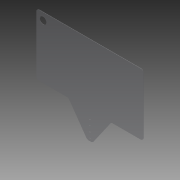
# Autodesk Inventor part: Funnel 2
Saved by Autodesk Inventor 2014 (Build 180170000, 170)
## iProperties
Created: 2014-01-07
Part Number: Funnel 2
Material: Polycarbonate, Clear
Document SubType Name: Modeling
Designer: Michael
Density: 1.2 g/cm^3
Appearance: Polycarbonate - Clear
Author: Michael
Autodesk Inventor part; units mm, degrees
ref_plane "YZ Plane" through (0, 0, 0) normal (1, 0, 0) x (0, 1, 0)
ref_plane "XZ Plane" through (0, 0, 0) normal (0, 1, 0) x (-1, 0, 0)
ref_plane "XY Plane" through (0, 0, 0) normal (0, 0, 1) x (1, 0, 0)
sketch "Sketch1" plane through (0, 0, 0) normal (0, 0, 1) x (1, 0, 0)
  line L0 (0, 0) -> (25.4, 0)
  line L1 (25.4, 0) -> (114.3, 127)
  line L2 (12.7, 0) -> (12.7, 419.1) construction
  line L3 (114.3, 127) -> (266.7, 127)
  line L4 (266.7, 127) -> (266.7, 419.1)
  line L5 (266.7, 419.1) -> (12.7, 419.1)
  circle A0 centre (12.7, 12.7) radius 2.0828
  circle A1 centre (12.7, 38.1) radius 2.0828
  circle A2 centre (12.7, 63.5) radius 2.0828
  circle A3 centre (12.7, 88.9) radius 2.0828
  line L6 (0, 0) -> (-88.9, 127)
  line L7 (-88.9, 127) -> (-241.3, 127)
  line L8 (-241.3, 127) -> (-241.3, 419.1)
  line L9 (-241.3, 419.1) -> (12.7, 419.1)
  dimension "d0" = 25.4
  dimension "d2" = 254
  dimension "d3" = 419.1
  dimension "d4" = 127
  dimension "d5" = 152.4
  dimension "d6" = 4.1656
  dimension "d7" = 12.7
  dimension "d10" = 25.4
  constraints: 20 end point, 4 centre point, 4 perpendicular, 3 symmetric about line, 1 horizontal, 1 midpoint, 1 point on line, 1 vertical, 6 other
  measures "d0" distance of L0.start L0.end
  measures "d2" distance between parallel lines of L2 L4
  measures "d3" distance from line of L2.start L5
  measures "d4" distance between parallel lines of L0 L3
  measures "d5" distance of L1.end L3.end
  measures "d6" diameter of A0
  measures "d7" distance from line of L0 A0.centre
  measures "d10" distance of A0.centre A1.centre
extrude "Extrusion1" add sketch "Sketch1" along normal blind 1.5875
fillet "Fillet1" radius 12.7 8 edges at (25.4, 0, 0.7937) (114.3, 127, 0.7937) (266.7, 127, 0.7937) (266.7, 419.1, 0.7937) (-241.3, 419.1, 0.7937) (-241.3, 127, 0.7937) (-88.9, 127, 0.7937) (0, 0, 0.7937)
sketch "Sketch2" plane through (0, 0, 1.5875) normal (0, 0, 1) x (1, 0, 0)
  line L0 (254, 419.1) -> (-228.6, 419.1) projected
  line L1 (-241.3, 406.4) -> (-241.3, 139.7) projected
  circle A0 centre (-209.55, 384.175) radius 15.875
  circle A1 centre (-165.1, 384.175) radius 15.875
  circle A2 centre (-120.65, 384.175) radius 15.875
  circle A3 centre (-76.2, 384.175) radius 15.875
  circle A4 centre (-31.75, 384.175) radius 15.875
  circle A5 centre (12.7, 384.175) radius 15.875
  circle A6 centre (57.15, 384.175) radius 15.875
  circle A7 centre (101.6, 384.175) radius 15.875
  circle A8 centre (146.05, 384.175) radius 15.875
  circle A9 centre (190.5, 384.175) radius 15.875
  circle A10 centre (234.95, 384.175) radius 15.875
  circle A11 centre (-209.55, 339.725) radius 15.875
  circle A12 centre (-165.1, 339.725) radius 15.875
  circle A13 centre (-120.65, 339.725) radius 15.875
  circle A14 centre (-76.2, 339.725) radius 15.875
  circle A15 centre (-31.75, 339.725) radius 15.875
  circle A16 centre (12.7, 339.725) radius 15.875
  circle A17 centre (57.15, 339.725) radius 15.875
  circle A18 centre (101.6, 339.725) radius 15.875
  circle A19 centre (146.05, 339.725) radius 15.875
  circle A20 centre (190.5, 339.725) radius 15.875
  circle A21 centre (234.95, 339.725) radius 15.875
  circle A22 centre (-209.55, 295.275) radius 15.875
  circle A23 centre (-165.1, 295.275) radius 15.875
  circle A24 centre (-120.65, 295.275) radius 15.875
  circle A25 centre (-76.2, 295.275) radius 15.875
  circle A26 centre (-31.75, 295.275) radius 15.875
  circle A27 centre (12.7, 295.275) radius 15.875
  circle A28 centre (57.15, 295.275) radius 15.875
  circle A29 centre (101.6, 295.275) radius 15.875
  circle A30 centre (146.05, 295.275) radius 15.875
  circle A31 centre (190.5, 295.275) radius 15.875
  circle A32 centre (234.95, 295.275) radius 15.875
  circle A33 centre (-209.55, 250.825) radius 15.875
  circle A34 centre (-165.1, 250.825) radius 15.875
  circle A35 centre (-120.65, 250.825) radius 15.875
  circle A36 centre (-76.2, 250.825) radius 15.875
  circle A37 centre (-31.75, 250.825) radius 15.875
  circle A38 centre (12.7, 250.825) radius 15.875
  circle A39 centre (57.15, 250.825) radius 15.875
  circle A40 centre (101.6, 250.825) radius 15.875
  circle A41 centre (146.05, 250.825) radius 15.875
  circle A42 centre (190.5, 250.825) radius 15.875
  circle A43 centre (234.95, 250.825) radius 15.875
  circle A44 centre (-209.55, 206.375) radius 15.875
  circle A45 centre (-165.1, 206.375) radius 15.875
  circle A46 centre (-120.65, 206.375) radius 15.875
  circle A47 centre (-76.2, 206.375) radius 15.875
  circle A48 centre (-31.75, 206.375) radius 15.875
  circle A49 centre (12.7, 206.375) radius 15.875
  circle A50 centre (57.15, 206.375) radius 15.875
  circle A51 centre (101.6, 206.375) radius 15.875
  circle A52 centre (146.05, 206.375) radius 15.875
  circle A53 centre (190.5, 206.375) radius 15.875
  circle A54 centre (234.95, 206.375) radius 15.875
  circle A55 centre (-209.55, 161.925) radius 15.875
  circle A56 centre (-165.1, 161.925) radius 15.875
  circle A57 centre (-120.65, 161.925) radius 15.875
  circle A58 centre (-76.2, 161.925) radius 15.875
  circle A59 centre (-31.75, 161.925) radius 15.875
  circle A60 centre (12.7, 161.925) radius 15.875
  circle A61 centre (57.15, 161.925) radius 15.875
  circle A62 centre (101.6, 161.925) radius 15.875
  circle A63 centre (146.05, 161.925) radius 15.875
  circle A64 centre (190.5, 161.925) radius 15.875
  circle A65 centre (234.95, 161.925) radius 15.875
  circle A66 centre (-209.55, 117.475) radius 15.875
  circle A67 centre (-165.1, 117.475) radius 15.875
  circle A68 centre (-120.65, 117.475) radius 15.875
  circle A69 centre (-76.2, 117.475) radius 15.875
  circle A70 centre (-31.75, 117.475) radius 15.875
  circle A71 centre (12.7, 117.475) radius 15.875
  circle A72 centre (57.15, 117.475) radius 15.875
  circle A73 centre (101.6, 117.475) radius 15.875
  circle A74 centre (146.05, 117.475) radius 15.875
  circle A75 centre (190.5, 117.475) radius 15.875
  circle A76 centre (234.95, 117.475) radius 15.875
  circle A77 centre (-209.55, 73.025) radius 15.875
  circle A78 centre (-165.1, 73.025) radius 15.875
  circle A79 centre (-120.65, 73.025) radius 15.875
  circle A80 centre (-76.2, 73.025) radius 15.875
  circle A81 centre (-31.75, 73.025) radius 15.875
  circle A82 centre (12.7, 73.025) radius 15.875
  circle A83 centre (57.15, 73.025) radius 15.875
  circle A84 centre (101.6, 73.025) radius 15.875
  circle A85 centre (146.05, 73.025) radius 15.875
  circle A86 centre (190.5, 73.025) radius 15.875
  circle A87 centre (234.95, 73.025) radius 15.875
  point P0 (0, 0)
  dimension "d18" = 31.75
  dimension "d19" = 34.925
  dimension "d20" = 31.75
  dimension "d23" = 44.45
  dimension "d26" = 44.45
  constraints: 88 centre point, 1 horizontal, 1 vertical, 174 other
  measures "d18" diameter of A0
  measures "d19" distance from line of L0 A0.centre
  measures "d20" distance from line of L1 A0.centre
  measures "d23" distance of A0.centre A1.centre
  measures "d26" distance of A0.centre A11.centre
extrude "Extrusion2" cut sketch "Sketch2" against normal blind 1.5875 contours A0
body "Solid1"
